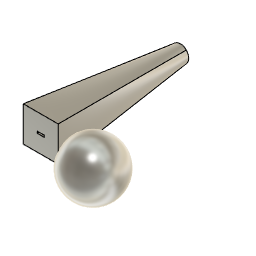
XSectionTest (Autodesk Fusion 360 design; units mm, degrees)
Autodesk Fusion 360 part; units mm, degrees
sketch "Sketch1" plane through (0, 0, 0) normal (0, 1, 0) x (1, 0, 0)
  line L0 (0, 0) -> (25, 0)
  line L1 (25, 0) -> (25, -25)
  line L2 (25, -25) -> (0, -25)
  line L3 (0, -25) -> (0, 0)
  line L4 (10, -13) -> (15, -13)
  line L5 (15, -13) -> (15, -11.6916)
  line L6 (15, -11.6916) -> (10, -11.6916)
  line L7 (10, -11.6916) -> (10, -13)
  dimension "d1" = 25
  dimension "d2" = 25
  constraint horizontal L0
  constraint vertical L1
  constraint horizontal L2
  constraint vertical L3
  constraint coincident L0.start L3.end
  constraint horizontal L4
  constraint vertical L5
  constraint horizontal L6
  constraint vertical L7
  measures "d1" distance of L0.start L2.end
  measures "d2" distance of L1.end L2.end
ref_plane "WorkPlane1" through (12.5, 100, 12.5) normal (0, 1, 0) x (1, 0, 0)
sketch "Sketch2" plane through (0, 100, 0) normal (0, 1, 0) x (1, 0, 0)
  circle A0 centre (12.5, -12.5) radius 6
  line L0 (25, -25) -> (0, -25)
  line L1 (25, 0) -> (25, -25)
  line L2 (0, 0) -> (25, 0)
  line L3 (0, -25) -> (25, 0) construction
  line L4 (0, 0) -> (25, -25) construction
  dimension "d4" = 12
  constraint coincident L0.end L3.start
  constraint coincident L1.start L2.end
  constraint coincident L2.start L4.start
  constraint coincident L0.start L1.end
  constraint coincident A0.centre L4
  constraint coincident A0.centre L3
  measures "d4" diameter of A0
loft "Loft1" add profiles "Sketch1", "Sketch2" section 1 contours L0 L1 L2 L3 | L4 L5 L6 L7 section 2 makes body 1
extrude "Extrude1" cut sketch "Sketch1" along normal through all contours L4 L5 L6 L7 bodies 1
sketch "Sketch9" plane through (0, 0, 0) normal (0, 0, 1) x (1, 0, 0)
  line L0 (0, 0) -> (0, 100)
  constraint coincident L0.start origin
  constraint vertical L0
sphere "SpherePrimitive2" add diameter 40 placed x (1, 0, 0) y (0, 1, 0) z (0, 0, 1) at (40, 10, 0) separate body makes body 2
